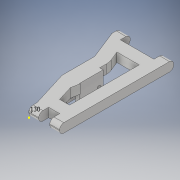
# Autodesk Inventor part: Part1
Saved by Autodesk Inventor 2018 (Build 220112000, 112)
## iProperties
Created: 2017-11-13
Part Number: Part1
Material: Generic
Document SubType Name: Modeling
Designer: Intel
Density: 1 g/cm^3
Appearance: Default
Author: Intel
Autodesk Inventor part; units mm, degrees
ref_plane "YZ Plane" through (0, 0, 0) normal (1, 0, 0) x (0, 1, 0)
ref_plane "XZ Plane" through (0, 0, 0) normal (0, 1, 0) x (-1, 0, 0)
ref_plane "XY Plane" through (0, 0, 0) normal (0, 0, 1) x (1, 0, 0)
sketch "Sketch1" plane through (0, 0, 0) normal (0, 1, 0) x (-1, 0, 0)
  line L0 (0, 0) -> (0, -88.265)
  line L1 (0, -88.265) -> (41.275, -88.265)
  line L2 (0, 0) -> (23.8125, 0)
  line L3 (32.4358, -34.29) -> (32.4358, -59.69)
  line L4 (41.275, -88.265) -> (41.275, -81.915)
  line L5 (23.8125, 0) -> (23.8125, -6.35)
  line L6 (23.8125, -6.35) -> (32.4358, -34.29)
  line L7 (32.4358, -59.69) -> (41.275, -81.915)
  line L8 (33.655, -88.265) -> (33.655, -80.645)
  line L9 (7.62, -88.265) -> (7.62, -80.645)
  line L10 (7.62, -80.645) -> (33.655, -80.645)
  line L11 (16.1925, 0) -> (16.1925, -7.62)
  line L12 (16.1925, -7.62) -> (7.62, -7.62)
  line L13 (7.62, -7.62) -> (7.62, 0)
  point P0 (32.4358, -46.99)
  dimension "d0" = 88.265
  dimension "d1" = 41.275
  dimension "d2" = 23.8125
  dimension "d3" = 41.275
  dimension "d4" = 32.4358
  dimension "d5" = 25.4
  dimension "d6" = 12.7
  dimension "d10" = 6.35
  dimension "d11" = 6.35
  dimension "d12" = 7.62
  dimension "d13" = 7.62
  dimension "d14" = 7.62
  dimension "d15" = 7.62
  dimension "d16" = 7.62
  dimension "d17" = 7.62
  constraints: 28 end point, 7 vertical, 4 perpendicular, 4 point on line, 1 coincident, 1 horizontal, 1 midpoint
  measures "d0" distance of L0.start L0.end
  measures "d1" distance of L0.end L1.end
  measures "d2" distance of L0.start L2.end
  measures "d3" distance from line of L1 point (32.436, -46.99)
  measures "d4" distance from line of L0 point (32.436, -46.99)
  measures "d5" distance of L3.start L3.end
  measures "d6" distance of L3.end point (32.436, -46.99)
  measures "d10" distance of L1.end L4.end
  measures "d11" distance of L2.end L5.end
  measures "d12" distance between parallel lines of L4 L8
  measures "d13" distance between parallel lines of L0 L9
  measures "d14" distance between parallel lines of L1 L10
  measures "d15" distance of L11.start L11.end
  measures "d16" distance between parallel lines of L11 L5
  measures "d17" distance between parallel lines of L0 L13
extrude "Extrusion1" add sketch "Sketch1" along normal blind 6.985 contours L2 L13 L12 L11 L5 L6 L3 L7 L4 L1 L8 L10 L9 L0
fillet "Fillet2" radius 3.175 12 edges at (-41.275, 3.4925, -81.915) (-32.4358, 3.4925, -59.69) (-32.4358, 3.4925, -34.29) (-23.8125, 3.4925, -6.35) (-3.81, 0, 0) (-3.81, 6.985, 0) (-20.0025, 0, 0) (-20.0025, 6.985, 0) (-37.465, 0, -88.265) (-37.465, 6.985, -88.265) (-3.81, 0, -88.265) (-3.81, 6.985, -88.265)
sketch "Sketch2" plane through (0, 6.985, 0) normal (0, 1, 0) x (1, 0, 0)
  line L0 (-7.62, 85.09) -> (0, 85.09) projected
  line L1 (-7.62, 85.09) -> (-7.62, 80.645) projected
  line L2 (-7.62, 80.645) -> (-33.655, 80.645) projected
  line L3 (-33.655, 80.645) -> (-33.655, 85.09) projected
  line L4 (-41.275, 85.09) -> (-33.655, 85.09) projected
  line L5 (-41.275, 85.09) -> (-41.275, 82.5232) projected
  arc A0 (-41.275, 82.5232) -> (-41.0502, 81.3499) centre (-38.1, 82.5232) ccw projected
  line L6 (-41.0502, 81.3499) -> (-32.6606, 60.2551) projected
  arc A1 (-32.4358, 59.0818) -> (-32.6606, 60.2551) centre (-35.6108, 59.0818) ccw projected
  line L7 (-32.4358, 59.0818) -> (-32.4358, 34.7688) projected
  arc A2 (-32.4358, 34.7688) -> (-32.2946, 33.8325) centre (-29.2608, 34.7688) ccw projected
  line L8 (-32.2946, 33.8325) -> (-23.9537, 6.8075) projected
  arc A3 (-23.8125, 5.8712) -> (-23.9537, 6.8075) centre (-26.9875, 5.8712) ccw projected
  line L9 (-23.8125, 5.8712) -> (-23.8125, 3.175) projected
  line L10 (-16.1925, 3.175) -> (-23.8125, 3.175) projected
  line L11 (-16.1925, 3.175) -> (-16.1925, 7.62) projected
  line L12 (-16.1925, 7.62) -> (-7.62, 7.62) projected
  line L13 (-7.62, 7.62) -> (-7.62, 3.175) projected
  line L14 (0, 3.175) -> (-7.62, 3.175) projected
  line L15 (0, 3.175) -> (0, 85.09) projected
  line L16 (-22.9108, 35.7265) -> (-22.9108, 59.0818)
  arc A4 (-22.9108, 59.0818) -> (-23.8099, 63.7752) centre (-35.6108, 59.0818) ccw
  line L17 (-23.8099, 63.7752) -> (-26.731, 71.12)
  line L18 (-26.731, 71.12) -> (-9.525, 71.12)
  line L19 (-9.525, 71.12) -> (-9.525, 17.145)
  line L20 (-9.525, 17.145) -> (-17.1759, 17.145)
  line L21 (-17.1759, 17.145) -> (-22.9108, 35.7265)
  line L22 (-32.4358, 59.0818) -> (-32.4358, 34.7688) projected
  line L23 (-32.4358, 53.8188) -> (-29.2608, 53.8188)
  line L24 (-29.2608, 53.8188) -> (-29.2608, 34.7688)
  line L25 (-29.2608, 34.7688) -> (-32.4358, 34.7688)
  line L26 (-32.4358, 34.7688) -> (-32.4358, 59.0818)
  line L27 (-19.7358, 54.7765) -> (-19.7358, 35.7265)
  line L28 (-19.7358, 35.7265) -> (-22.9108, 35.7265)
  line L29 (-19.7358, 35.7265) -> (-20.8902, 29.1796)
  line L30 (-22.9108, 35.7265) -> (-22.9108, 54.7765)
  line L31 (-22.9108, 54.7765) -> (-19.7358, 54.7765)
  point P0 (0, 0)
  dimension "d19" = 9.525
  dimension "d25" = 3.175
  dimension "d26" = 3.175
  dimension "d28" = 80
  dimension "d44" = 19.05
  dimension "d45" = 19.05
  dimension "d46" = 19.05
  constraints: 31 end point, 3 perpendicular, 2 parallel, 2 point on circle, 2 point on line, 1 centre point, 1 horizontal, 1 vertical, 6 other
  measures "d19" distance between parallel lines of L7 L16
  measures "d25" distance of L7.end L24.end
  measures "d26" distance of L16.start L27.end
  measures "d28" angle of L28 L29
  measures "d44" distance between parallel lines of L25 L23
  measures "d45" distance of L16.start L30.end
  measures "d46" distance from line of L28 L27.start
extrude "Extrusion2" cut sketch "Sketch2" against normal blind 6.985 contours L16 L31 L27 L28 | L16 A4 L17 L18 L19 L20 L21 L29 L27 L31
sketch "Sketch3" plane through (0, 6.985, 0) normal (0, 1, 0) x (1, 0, 0)
  line L0 (-32.4358, 59.0818) -> (-32.4358, 34.7688) projected
  line L1 (-32.4358, 59.0818) -> (-29.2608, 59.0818)
  line L2 (-29.2608, 59.0818) -> (-29.2608, 34.7688)
  line L3 (-29.2608, 34.7688) -> (-32.4358, 34.7688)
  line L4 (-32.4358, 34.7688) -> (-32.4358, 59.0818)
  line L5 (-20.8902, 29.1796) -> (-17.1759, 17.145) projected
  line L6 (-23.4823, 59.0818) -> (-22.9108, 59.0818)
  line L7 (-22.9108, 59.0818) -> (-22.9108, 35.7265)
  line L8 (-22.9108, 35.7265) -> (-23.4823, 35.7265)
  line L9 (-23.4823, 35.7265) -> (-23.4823, 59.0818)
  point P0 (0, 0)
  dimension "d22" = 3.175
  dimension "d24" = 5.7785
  constraints: 16 end point, 4 parallel, 2 horizontal, 2 perpendicular, 1 point on line
  measures "d22" distance of L0.end L2.end
  measures "d24" distance between parallel lines of L2 L9
sketch "Sketch4" plane through (0, 6.985, 0) normal (0, 1, 0) x (1, 0, 0)
  line L0 (-32.4358, 53.8188) -> (-29.2608, 53.8188)
  line L1 (-29.2608, 53.8188) -> (-29.2608, 34.7688)
  line L2 (-29.2608, 34.7688) -> (-32.4358, 34.7688)
  line L3 (-32.4358, 34.7688) -> (-32.4358, 53.8188)
  line L4 (-20.2438, 59.0818) -> (-20.2438, 35.7265) projected
  line L5 (-20.2438, 53.8188) -> (-23.4188, 53.8188)
  line L6 (-23.4188, 53.8188) -> (-23.4188, 35.7265)
  line L7 (-23.4188, 35.7265) -> (-20.2438, 35.7265)
  line L8 (-20.2438, 35.7265) -> (-20.2438, 59.0818)
  point P0 (0, 0)
  dimension "d29" = 3.175
  dimension "d30" = 3.175
  dimension "d43" = 19.05
  constraints: 16 end point, 4 parallel, 2 collinear, 2 horizontal, 2 perpendicular, 1 coincident, 1 point on line
  measures "d29" distance of L1.end L2.end
  measures "d30" distance of L4.end L6.end
  measures "d43" distance between parallel lines of L0 L2
extrude "Extrusion3" add sketch "Sketch4" against normal blind 17.78
sketch "Sketch5" plane through (-32.4358, 6.985, -59.0818) normal (-1, 0, 0) x (0, 0, 1)
  circle A0 centre (20.757, -14.732) radius 1.27
  line L0 (0, 0) -> (24.313, 0) projected
  circle A1 centre (14.5613, -12.446) radius 1.27
  circle A2 centre (8.3655, -10.16) radius 1.27
  line L1 (24.313, -6.985) -> (24.313, -17.78) projected
  line L2 (20.757, -14.732) -> (8.3655, -10.16) construction
  point P0 (59.0818, -6.985)
  dimension "d33" = 2.54
  dimension "d34" = 14.732
  dimension "d35" = 2.54
  dimension "d36" = 6.604
  dimension "d37" = 2.54
  dimension "d38" = 6.604
  dimension "d39" = 10.16
  dimension "d40" = 3.556
  constraints: 3 centre point, 2 end point, 1 midpoint
  measures "d33" diameter of A0
  measures "d34" distance from line of L0 L2.start
  measures "d35" diameter of A1
  measures "d36" distance of A1.centre L2.start
  measures "d37" diameter of A2
  measures "d38" distance of L2.end A1.centre
  measures "d39" distance from line of L0 L2.end
  measures "d40" distance from line of L1 L2.start
extrude "Extrusion4" cut sketch "Sketch5" against normal blind 25.4
sketch "Sketch6" plane through (-23.8125, 0, -5.8712) normal (-1, 0, 0) x (0, 0, 1)
  circle A0 centre (2.5695, 3.5161) radius 1.651
  point P0 (5.8712, 0)
  dimension "d47" = 3.302
  constraints: 1 centre point
  measures "d47" diameter of A0
equation "\"d38\" = d36"
body "Solid1"
